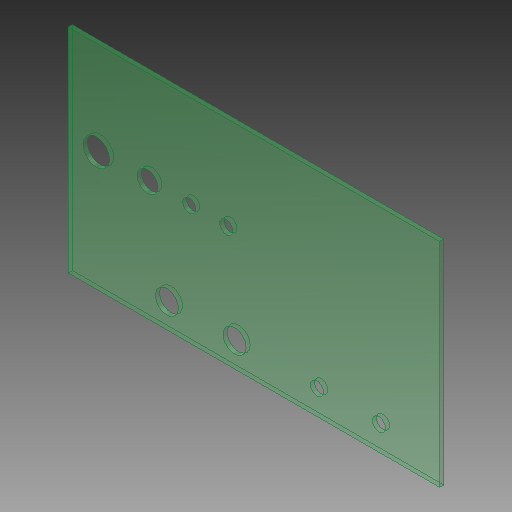
# Autodesk Inventor part: sb_front_back
Saved by Autodesk Inventor 2018.1 (Build 221171000, 171)
## iProperties
Created: 2017-08-17
Part Number: sb_front_back
Material: PVC-Piping
Document SubType Name: Modeling
Designer: Tom
Density: 1.4 g/cm^3
Appearance: Clear - Green 1
Author: Tom
Autodesk Inventor part; units mm, degrees
ref_plane "YZ Plane" through (0, 0, 0) normal (1, 0, 0) x (0, 1, 0)
ref_plane "XZ Plane" through (0, 0, 0) normal (0, 1, 0) x (-1, 0, 0)
ref_plane "XY Plane" through (0, 0, 0) normal (0, 0, 1) x (1, 0, 0)
sketch "Sketch1" plane through (0, 0, 0) normal (0, 0, 1) x (1, 0, 0)
  line L0 (-225, -129) -> (225, -129)
  line L1 (225, -129) -> (225, 129)
  line L2 (225, 129) -> (-225, 129)
  line L3 (-225, 129) -> (-225, -129)
  line L4 (-225, -129) -> (225, 129) construction
  line L5 (225, -129) -> (-225, 129) construction
  point P0 (0, 0)
  dimension "d0" = 450
  dimension "d1" = 258
  constraints: 12 end point, 2 midpoint, 2 parallel, 1 horizontal, 1 perpendicular
  measures "d0" distance of L2.end L1.end
  measures "d1" distance of L1.end L0.end
extrude "Extrusion1" add sketch "Sketch1" along normal mid plane 5
sketch "Sketch2" plane through (0, 0, 2.5) normal (0, 0, 1) x (1, 0, 0)
  circle A0 centre (-105.5, -99.5) radius 19.5 construction
  line L0 (-225, -129) -> (225, -129) construction
  line L1 (-225, 129) -> (-225, -129) construction
  circle A1 centre (-23.5, -99.5) radius 19.5 construction
  circle A2 centre (76.5, -99.5) radius 12.5 construction
  circle A3 centre (151.5, -99.5) radius 12.5 construction
  circle A4 centre (-191, 15) radius 24 construction
  circle A5 centre (-129, 15) radius 18 construction
  circle A6 centre (-78.5, 15) radius 12.5 construction
  circle A7 centre (-33.5, 15) radius 12.5 construction
  circle A8 centre (-191, 15) radius 16
  circle A9 centre (-129, 15) radius 12.5
  circle A10 centre (-78.5, 15) radius 8
  circle A11 centre (-33.5, 15) radius 8
  circle A12 centre (-105.5, -99.5) radius 14
  circle A13 centre (-23.5, -99.5) radius 14
  circle A14 centre (76.5, -99.5) radius 8
  circle A15 centre (151.5, -99.5) radius 8
  point P0 (0, 0)
  dimension "d4" = 39
  dimension "d5" = 29.5
  dimension "d6" = 119.5
  dimension "d7" = 39
  dimension "d8" = 25
  dimension "d9" = 25
  dimension "d10" = 48
  dimension "d11" = 36
  dimension "d12" = 25
  dimension "d13" = 25
  dimension "d14" = 29.5
  dimension "d15" = 29.5
  dimension "d16" = 29.5
  dimension "d17" = 144
  dimension "d18" = 144
  dimension "d19" = 144
  dimension "d20" = 144
  dimension "d21" = 82
  dimension "d22" = 100
  dimension "d23" = 75
  dimension "d24" = 34
  dimension "d25" = 62
  dimension "d26" = 50.5
  dimension "d27" = 45
  dimension "d28" = 32
  dimension "d29" = 25
  dimension "d30" = 16
  dimension "d31" = 16
  dimension "d32" = 28
  dimension "d33" = 28
  dimension "d34" = 16
  dimension "d35" = 16
  constraints: 16 centre point, 8 coincident
  measures "d4" diameter of A0
  measures "d5" distance from line of L0 A0.centre
  measures "d6" distance from line of L1 A0.centre
  measures "d7" diameter of A1
  measures "d8" diameter of A2
  measures "d9" diameter of A3
  measures "d10" diameter of A4
  measures "d11" diameter of A5
  measures "d12" diameter of A6
  measures "d13" diameter of A7
  measures "d14" distance from line of L0 A1.centre
  measures "d15" distance from line of L0 A2.centre
  measures "d16" distance from line of L0 A3.centre
  measures "d17" distance from line of L0 A4.centre
  measures "d18" distance from line of L0 A5.centre
  measures "d19" distance from line of L0 A6.centre
  measures "d20" distance from line of L0 A7.centre
  measures "d21" distance of A1.centre A0.centre
  measures "d22" distance of A2.centre A1.centre
  measures "d23" distance of A3.centre A2.centre
  measures "d24" distance from line of L1 A4.centre
  measures "d25" distance of A5.centre A4.centre
  measures "d26" distance of A6.centre A5.centre
  measures "d27" distance of A6.centre A7.centre
  measures "d28" diameter of A8
  measures "d29" diameter of A9
  measures "d30" diameter of A10
  measures "d31" diameter of A11
  measures "d32" diameter of A12
  measures "d33" diameter of A13
  measures "d34" diameter of A14
  measures "d35" diameter of A15
extrude "Extrusion2" cut sketch "Sketch2" against normal blind 5
equation "\"d0\" = boxw"
equation "\"d1\" = boxh"
equation "\"d2\" = pvct"
equation "\"d4\" = waterouter"
equation "\"d6\" = 0.5 * waterouter + distsidewater"
equation "\"d7\" = airoutouter"
equation "\"d8\" = pumpouter"
equation "\"d9\" = pumpouter"
equation "\"d10\" = diaphouter"
equation "\"d11\" = diaetapeouter"
equation "\"d12\" = dialoadouter"
equation "\"d13\" = dialoadouter"
equation "\"d21\" = distbubblewater"
equation "\"d22\" = distpumpbubble"
equation "\"d23\" = distpumps"
equation "\"d28\" = diaph"
equation "\"d29\" = diaetape"
equation "\"d30\" = pumpinner"
equation "\"d31\" = pumpinner"
equation "\"d32\" = waterinner"
equation "\"d33\" = airoutinner"
equation "\"d34\" = pumpinner"
equation "\"d35\" = pumpinner"
equation "\"d36\" = pvct"
equation "\"solhole\" = 3"
equation "\"solholespacing\" = 16"
equation "\"ssolw\" = 63"
equation "\"bsoll\" = 126"
equation "\"bsolw\" = 91"
equation "\"bsolh\" = 126"
equation "\"tapl\" = 31"
equation "\"tl\" = 32"
equation "\"eloboww\" = 25"
equation "\"pvct\" = 5"
equation "\"boxw\" = 450"
equation "\"boxh\" = 258"
equation "\"supporth\" = 15"
equation "\"play\" = 0.5"
equation "\"pcbw\" = 76"
equation "\"arw\" = 54"
equation "\"pcbl\" = 86"
equation "\"arl\" = 102"
equation "\"psuh\" = 85"
equation "\"pcbh\" = 46"
equation "\"screenl\" = 115"
equation "\"screenw\" = 197"
equation "\"seph\" = 105"
equation "\"diapowerouter\" = 25"
equation "\"dialoadouter\" = 25"
equation "\"diaetapeouter\" = 36"
equation "\"diaphouter\" = 48"
equation "\"diaload\" = 16"
equation "\"diaetape\" = 25"
equation "\"diaph\" = 32"
equation "\"distbubblewater\" = 82"
equation "\"diapower\" = 16"
equation "\"distpumpbubble\" = 100"
equation "\"waterinner\" = 28"
equation "\"distpumps\" = 75"
equation "\"airoutouter\" = 39"
equation "\"airoutinner\" = 28"
equation "\"pumpouter\" = 25"
equation "\"waterouter\" = 39"
equation "\"pumpinner\" = 16"
equation "\"airinouter\" = 39"
equation "\"airininner\" = 28"
equation "\"distsidewater\" = 100"
body "Solid1"
